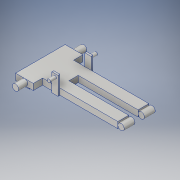
# Autodesk Inventor part: elevbase
Saved by Autodesk Inventor 2016 (Build 200138000, 138)
## iProperties
Created: 2018-01-09
Part Number: elevbase
Material: Aluminum 6061
Document SubType Name: Modeling
Designer: New User
Density: 2.7 g/cm^3
Appearance: Aluminum - Flat
Mass: 29172.4 g
Surface Area: 6754.29 cm^2
Volume: 10804.6 cm^3
Author: New User
Autodesk Inventor part; units mm, degrees
ref_plane "YZ Plane" through (0, 0, 0) normal (1, 0, 0) x (0, 1, 0)
ref_plane "XZ Plane" through (0, 0, 0) normal (0, 1, 0) x (-1, 0, 0)
ref_plane "XY Plane" through (0, 0, 0) normal (0, 0, 1) x (1, 0, 0)
sketch "Sketch1" plane through (0, 0, 0) normal (0, 1, 0) x (-1, 0, 0)
  line L0 (0, 0) -> (-145.4185, 0)
  line L1 (-145.4185, -406.4) -> (0, -406.4)
  line L2 (0, -406.4) -> (0, 0)
  line L3 (-145.4185, 0) -> (-145.4185, -76.2)
  line L4 (-145.4185, -76.2) -> (-762, -76.2)
  line L5 (-762, -330.2) -> (-145.4185, -330.2)
  line L6 (-145.4185, -330.2) -> (-145.4185, -406.4)
  line L7 (-762, -165.1) -> (-272.4185, -165.1)
  line L8 (-272.4185, -165.1) -> (-272.4185, -241.3)
  line L9 (-272.4185, -241.3) -> (-762, -241.3)
  line L10 (-762, -76.2) -> (-762, -165.1)
  line L11 (-762, -241.3) -> (-762, -330.2)
  dimension "d0" = 406.4
  dimension "d8" = 76.2
  dimension "d9" = 76.2
  dimension "d10" = 88.9
  dimension "d11" = 88.9
  dimension "d23" = 762
  dimension "d24" = 762
  constraints: 24 end point, 5 parallel, 5 perpendicular, 2 horizontal, 2 point on line, 1 vertical
  measures "d0" distance of L1.end L0.start
  measures "d8" distance of L0.end L3.end
  measures "d9" distance of L1.start L5.end
  measures "d10" distance of L9.end L5.start
  measures "d11" distance of L4.end L7.start
  measures "d23" distance between parallel lines of L2 L10
  measures "d24" distance between parallel lines of L2 L11
extrude "Extrusion1" add sketch "Sketch1" along normal blind 50.8
sketch "Sketch2" plane through (0, 0, 0) normal (0, 0, 1) x (1, 0, 0)
  circle A0 centre (75.6822, 25.4) radius 25.4
  line L0 (0, 50.8) -> (762, 50.8) projected
  line L1 (0, 0) -> (0, 50.8) projected
  dimension "d40" = 75.6822
  constraints: 1 centre point, 1 tangent
  measures "d40" distance from line of L1 A0.centre
extrude "Extrusion2" add sketch "Sketch2" along normal blind 76.2 and the other way blind 482.6
sketch "Sketch3" plane through (145.4185, 0, -76.2) normal (0, 0, 1) x (1, 0, 0)
  line L0 (616.5815, 50.8) -> (127, 50.8) projected
  line L1 (0, 0) -> (616.5815, 0) projected
  line L2 (142.6302, 0) -> (168.0302, 0)
  line L3 (142.6302, 149.0545) -> (91.8302, 149.0545)
  line L4 (91.8302, 149.0545) -> (91.8302, 0)
  line L5 (91.8302, 0) -> (142.6302, 0)
  line L6 (142.6302, 0) -> (142.6302, 149.0545)
  point P0 (-145.4185, 0)
  point P1 (168.0302, 50.8)
  point P2 (117.2302, 0)
  constraints: 10 end point, 4 point on line, 2 parallel, 1 horizontal, 1 perpendicular
extrude "Extrusion3" add sketch "Sketch3" along normal blind 15.875
sketch "Sketch8" plane through (272.4185, 0, -241.3) normal (0, 0, 1) x (1, 0, 0)
  circle A0 centre (515.321, 25.4) radius 25.7395
  point P0 (-272.4185, 0)
  constraints: 1 centre point
extrude "Extrusion8" add sketch "Sketch8" along normal blind 165.1 and the other way blind 88.9
sketch "Sketch4" plane through (762, 0, -330.2) normal (0, 0, -1) x (-1, 0, 0)
  line L0 (448.5513, 0) -> (448.5513, 149.0545) projected
  line L1 (443.5591, 50.8) -> (499.3513, 50.8) projected
  line L2 (448.5513, 149.0545) -> (499.3513, 149.0545) projected
  line L3 (473.9513, 149.0545) -> (499.3513, 149.0545)
  line L4 (499.3513, 0) -> (524.7513, 0)
  line L5 (0, 0) -> (616.5815, 0) projected
  line L6 (448.5513, 0) -> (468.7254, 0)
  line L7 (473.9513, 0) -> (524.7513, 0)
  line L8 (524.7513, 0) -> (524.7513, 149.0545)
  line L9 (524.7513, 149.0545) -> (473.9513, 149.0545)
  line L10 (473.9513, 149.0545) -> (473.9513, 0)
  point P0 (762, 0)
  constraints: 14 end point, 3 point on line, 2 parallel, 1 collinear, 1 horizontal, 1 perpendicular, 1 other
extrude "Extrusion4" add sketch "Sketch4" along normal blind 15.875 contours L10 L2 L9 L8 L4 L5
sketch "Sketch9" plane through (272.4185, 0, -165.1) normal (1, 0, 0) x (0, 0, -1)
  line L0 (76.2, -11.7975) -> (0, -11.7975)
  line L1 (0, -11.7975) -> (0, 62.1226)
  line L2 (0, 62.1226) -> (76.2, 62.1226)
  line L3 (76.2, 62.1226) -> (76.2, -11.7975)
  point P0 (-165.1, 0)
  point P1 (76.2, 0)
  point P2 (0, 50.8)
  constraints: 8 end point, 2 parallel, 1 horizontal, 1 perpendicular
extrude "Extrusion9" cut sketch "Sketch9" along normal blind 844.55
sketch "Sketch5" plane through (762, 0, -346.075) normal (0, 0, -1) x (-1, 0, 0)
  circle A0 centre (499.3513, 123.6545) radius 12.7
  line L0 (448.5513, 149.0545) -> (499.3513, 149.0545) projected
  line L1 (499.3513, 0) -> (499.3513, 149.0545) projected
  point P0 (762, 0)
  dimension "d25" = 25.4
  dimension "d35" = 25.4
  dimension "d36" = 0
  constraints: 1 centre point
  measures "d25" diameter of A0
  measures "d35" distance from line of L0 A0.centre
  measures "d36" distance from line of L1 A0.centre
extrude "Extrusion5" add sketch "Sketch5" along normal blind 50.8
sketch "Sketch6" plane through (145.4185, 0, -60.325) normal (0, 0, 1) x (1, 0, 0)
  circle A0 centre (117.2302, 123.6545) radius 12.7
  line L0 (168.0302, 149.0545) -> (117.2302, 149.0545) projected
  line L1 (168.0302, 0) -> (168.0302, 149.0545) projected
  point P0 (-145.4185, 0)
  dimension "d26" = 25.4
  dimension "d38" = 25.4
  dimension "d39" = 50.8
  constraints: 1 centre point
  measures "d26" diameter of A0
  measures "d38" distance from line of L0 A0.centre
  measures "d39" distance from line of L1 A0.centre
extrude "Extrusion6" add sketch "Sketch6" along normal blind 50.8
sketch "Sketch10" plane through (0, 0, 0) normal (0, -1, 0) x (1, 0, 0)
  line L0 (0, -406.4) -> (0, 0) projected
  line L1 (0, -330.2) -> (36.7628, -330.2)
  line L2 (36.7628, -330.2) -> (36.7628, -76.2)
  line L3 (36.7628, -76.2) -> (0, -76.2)
  line L4 (0, -76.2) -> (0, -330.2)
  constraints: 8 end point, 2 parallel, 1 horizontal, 1 perpendicular, 1 point on line
extrude "Extrusion10" add sketch "Sketch10" along normal blind 82.55
body "Solid1"
